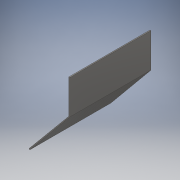
# Autodesk Inventor part: Cabin front panel
Saved by Autodesk Inventor 2019 (Build 230136000, 136)
## iProperties
Created: 2019-08-28
Part Number: Cabin front panel
Material: Steel, Mild
Document SubType Name: Modeling
Designer: DIBYOJYOTI
Density: 7.85 g/cm^3
Appearance: Semi-Polished
Mass: 52.631 g
Surface Area: 148.144 cm^2
Volume: 6.70458 cm^3
Author: DIBYOJYOTI
Autodesk Inventor part; units mm, degrees
ref_plane "YZ Plane" through (0, 0, 0) normal (1, 0, 0) x (0, 1, 0)
ref_plane "XZ Plane" through (0, 0, 0) normal (0, 1, 0) x (-1, 0, 0)
ref_plane "XY Plane" through (0, 0, 0) normal (0, 0, 1) x (1, 0, 0)
sketch "Sketch1" plane through (0, 0, 0) normal (0, 0, 1) x (1, 0, 0)
  line L0 (199.6028, -45.2691) -> (199.6028, -78.088)
  line L1 (199.6028, -78.088) -> (161.4068, -124)
  line L2 (199.6028, -45.2691) -> (200.6028, -45.2691)
  line L3 (200.6028, -45.2691) -> (200.6028, -78.088)
  line L4 (161.4068, -124) -> (162.1755, -124.6395)
  line L5 (162.1755, -124.6395) -> (200.6028, -78.088)
  point P0 (0, 0)
  dimension "d0" = 1
  dimension "d1" = 90
  dimension "d2" = 1
  dimension "d5" = 32.8188
  dimension "d6" = 60.3631
  dimension "d7" = 140.242
  constraints: 12 end point, 1 horizontal, 1 vertical
  measures "d0" distance of L0.start L2.end
  measures "d1" angle of L2 L3
  measures "d2" distance of L1.end L4.end
  measures "d5" distance of L2.end L3.end
  measures "d6" distance of L4.end L3.end
  measures "d7" angle of L0 L1
extrude "Extrusion1" add sketch "Sketch1" along normal blind 78
body "Solid1"
